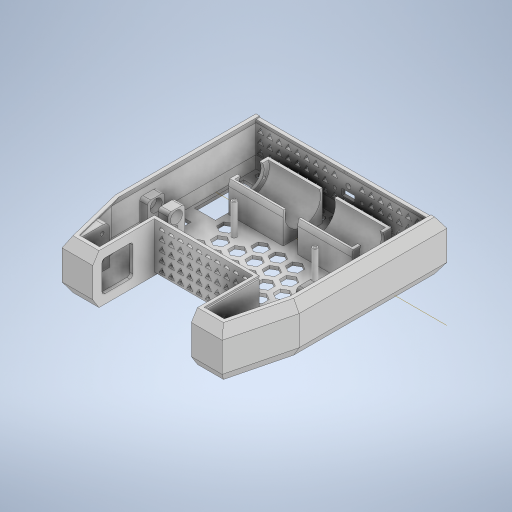
# Autodesk Inventor part: Bot v2 bottom
Saved by Autodesk Inventor 2024 (Build 280153000, 153)
## iProperties
Created: 2023-10-31
Part Number: Bot v2 bottom
Material: Generic
Document SubType Name: Modeling
Designer: CJ110
Density: 1 g/cm^3
Appearance: Default
Mass: 342.153 g
Surface Area: 1832.33 cm^2
Volume: 342.153 cm^3
Author: CJ110
## iProperties of the stored document Bot v2 bottom_3DPrint.ipt
Created: 2023-11-01
Part Number: Bot v2 bottom_3DPrint
Material: Generic
Document SubType Name: Modeling
Designer: CJ110
Density: 1 g/cm^3
Appearance: Default
Author: CJ110
Autodesk Inventor part; units mm, degrees
(part 1 of 3)
sketch "Sketch1" plane through (0, 0, 0) normal (0, 1, 0) x (-1, 0, 0)
  line L0 (0, 0) -> (152.4, 0)
  line L1 (152.4, 0) -> (152.4, 196.85)
  line L2 (152.4, 196.85) -> (0, 196.85)
  line L3 (0, 196.85) -> (0, 0)
  line L4 (152.4, 196.85) -> (215.9, 180.975)
  line L5 (215.9, 180.975) -> (215.9, 149.225)
  line L6 (215.9, 149.225) -> (152.4, 149.225)
  line L7 (152.4, 47.625) -> (215.9, 47.625)
  line L8 (215.9, 47.625) -> (215.9, 15.875)
  line L9 (215.9, 15.875) -> (152.4, 0)
  dimension "Bot_Main_Length" = 152.4
  dimension "Bot_Width" = 196.85
  dimension "Weapon_Support_Depth" = 63.5
  dimension "Weapon_Width" = 101.6
  dimension "d4" = 31.75
  dimension "d5" = 31.75
  constraints: 20 end point, 4 point on line, 3 parallel, 2 perpendicular, 1 equal length, 1 horizontal, 1 vertical
  measures "Bot_Main_Length" distance of L2.end L1.end
  measures "Bot_Width" distance of L0.end L1.end
  measures "Weapon_Support_Depth" distance between parallel lines of L1 L5
  measures "Weapon_Width" distance between parallel lines of L7 L6
  measures "d4" distance of L4.end L5.end
  measures "d5" distance of L7.end L8.end
extrude "Extrusion1" add sketch "Sketch1" along normal blind 50.8
chamfer "Chamfer1" distance 6.35 distance2 10.16 7 edges at (-76.2, 50.8, 196.85) (-184.15, 50.8, 188.9125) (0, 50.8, 98.425) (-76.2, 50.8, 0) (-184.15, 50.8, 7.9375) (-215.9, 50.8, 31.75) (-215.9, 50.8, 165.1) measured on face at (-215.4, 50.8, 165.1) measured on face at (-0.5, 50.8, 98.425) measured on face at (-184.0287, 50.8, 188.4274) measured on face at (-76.2, 50.8, 0.5) measured on face at (-76.2, 50.8, 196.35) measured on face at (-215.4, 50.8, 31.75) measured on face at (-184.0287, 50.8, 8.4226)
chamfer "Chamfer2" distance 6.35 distance2 10.16 7 edges at (-76.2, 0, 196.85) (-184.15, 0, 188.9125) (-215.9, 0, 165.1) (-184.15, 0, 7.9375) (-215.9, 0, 31.75) (-76.2, 0, 0) (0, 0, 98.425) measured on face at (-215.4, 0, 165.1) measured on face at (-184.0287, 0, 188.4274) measured on face at (-76.2, 0, 196.35) measured on face at (-76.2, 0, 0.5) measured on face at (-0.5, 0, 98.425) measured on face at (-184.0287, 0, 8.4226) measured on face at (-215.4, 0, 31.75)
shell "Shell1" thickness 3.175 removed faces 1 at (-55.033333, 50.8, 115.358333)
sketch "Sketch2" plane through (-151.401646, 3.175, 188.740264) normal (0, 1, 0) x (1, 0, 0)
  line L0 (11.701646, 3.175) -> (62.501646, 3.175)
  line L1 (62.501646, 3.175) -> (62.501646, 13.97)
  line L2 (62.501646, 13.97) -> (11.701646, 13.97)
  line L3 (11.701646, 13.97) -> (11.701646, 3.175)
  line L4 (76.61691, 3.175) -> (127.41691, 3.175)
  line L5 (127.41691, 3.175) -> (127.41691, 24.765)
  line L6 (127.41691, 24.765) -> (76.61691, 24.765)
  line L7 (76.61691, 24.765) -> (76.61691, 3.175)
  line L8 (143.29191, 0) -> (143.29191, 180.630527)
  line L9 (0, 0) -> (143.29191, 0)
  line L10 (2.176646, 36.340264) -> (2.176646, 144.290264)
  line L11 (2.176646, 90.315264) -> (141.307535, 90.315264) construction
  line L12 (141.307535, 178.646152) -> (141.307535, 1.984375) construction
  line L13 (-56.388618, 36.340264) -> (-56.388618, 14.097154)
  line L14 (-56.388618, 14.097154) -> (0, 0)
  line L15 (0, 0) -> (143.29191, 0)
  line L16 (143.29191, 0) -> (143.29191, 180.630527)
  line L17 (143.29191, 180.630527) -> (0, 180.630527)
  line L18 (0, 180.630527) -> (-56.388618, 166.533373)
  line L19 (-56.388618, 166.533373) -> (-56.388618, 144.290264)
  line L20 (-56.388618, 144.290264) -> (2.176646, 144.290264)
  line L21 (2.176646, 144.290264) -> (2.176646, 36.340264)
  line L22 (2.176646, 36.340264) -> (-56.388618, 36.340264)
  line L23 (11.701646, 177.455527) -> (62.501646, 177.455527)
  line L24 (62.501646, 177.455527) -> (62.501646, 166.660527)
  line L25 (62.501646, 166.660527) -> (11.701646, 166.660527)
  line L26 (11.701646, 166.660527) -> (11.701646, 177.455527)
  line L27 (76.61691, 177.455527) -> (127.41691, 177.455527)
  line L28 (127.41691, 177.455527) -> (127.41691, 155.865527)
  line L29 (127.41691, 155.865527) -> (76.61691, 155.865527)
  line L30 (76.61691, 155.865527) -> (76.61691, 177.455527)
  line L31 (102.01691, 24.765) -> (102.01691, 3.175) construction
  line L32 (37.101646, 13.97) -> (37.101646, 3.175) construction
  point P0 (151.401646, 188.740264)
  dimension "d15" = 21.59
  dimension "d16" = 50.8
  dimension "d17" = 50.8
  dimension "d19" = 3.175
  dimension "d21" = 10.795
  dimension "d165" = 41.275
  dimension "d166" = 34.925
  constraints: 38 end point, 8 symmetric about line, 6 midpoint, 4 parallel, 2 horizontal, 2 perpendicular, 1 collinear
  measures "d15" distance between parallel lines of L6 L4
  measures "d16" distance between parallel lines of L3 L1
  measures "d17" distance between parallel lines of L7 L5
  measures "d19" distance between parallel lines of L9 L4
  measures "d21" distance between parallel lines of L0 L2
  measures "d165" distance between parallel lines of L31 L8
  measures "d166" distance between parallel lines of L10 L32
extrude "Extrusion2" cut sketch "Sketch2" against normal through all contours L3 L2 L1 L0 | L7 L6 L5 L4 | L23 L24 L25 L26 | L27 L28 L29 L30
sketch "Sketch3" plane through (0, 40.64, 196.85) normal (1, 0, 0) x (0, 0, -1)
  line L0 (190.5, 10.16) -> (6.35, 10.16)
  line L1 (6.35, 10.16) -> (0, 0)
  line L2 (0, 0) -> (196.85, 0)
  line L3 (190.5, 10.16) -> (196.85, 0)
  line L4 (10.094111, 10.16) -> (8.109736, 6.985)
  line L5 (8.109736, 6.985) -> (188.740264, 6.985)
  line L6 (186.755889, 10.16) -> (188.740264, 6.985)
  point P0 (196.85, -40.64)
  dimension "d24" = 3.175
  dimension "d25" = 3.175
  dimension "d26" = 3.175
  constraints: 6 end point, 2 parallel, 2 point on line, 1 horizontal
  measures "d24" distance between parallel lines of L1 L4
  measures "d25" distance between parallel lines of L0 L5
  measures "d26" distance between parallel lines of L3 L6
extrude "Extrusion3" cut sketch "Sketch3" against normal up to surface contours L6 L5 L4 L0 surface through (-5.867395, 44.037253, 147.6375) normal (0.8479983, 0.5299989, 0)
sketch "Sketch4" plane through (-149.225, 3.175, 44.45) normal (1, 0, 0) x (0, 0, -1)
  line L0 (-144.290264, 44.45) -> (-142.305889, 47.625)
  line L1 (-142.305889, 47.625) -> (-146.05, 47.625)
  line L2 (-146.05, 47.625) -> (-152.4, 37.465)
  line L3 (-152.4, 37.465) -> (44.45, 37.465)
  line L4 (38.1, 47.625) -> (44.45, 37.465)
  line L5 (38.1, 47.625) -> (34.355889, 47.625)
  line L6 (34.355889, 47.625) -> (36.340264, 44.45)
  line L7 (36.340264, 44.45) -> (-144.290264, 44.45)
  line L8 (0, 0) -> (-107.95, 0)
  line L9 (0, 0) -> (0, 47.625)
  line L10 (-107.95, 47.625) -> (0, 47.625)
  line L11 (-107.95, 0) -> (-107.95, 47.625)
  line L12 (0, 46.0375) -> (-107.95, 46.0375)
  line L13 (-106.3625, 46.0375) -> (-106.3625, 44.45)
  line L14 (-1.5875, 46.0375) -> (-1.5875, 44.45)
  point P0 (44.45, -3.175)
  point P1 (-107.95, 44.45)
  point P2 (0, 44.45)
  dimension "d29" = 1.5875
  dimension "d30" = 1.5875
  dimension "d31" = 1.5875
  constraints: 6 end point, 6 point on line, 3 perpendicular
  measures "d29" distance between parallel lines of L10 L12
  measures "d30" distance between parallel lines of L11 L13
  measures "d31" distance between parallel lines of L9 L14
extrude "Extrusion4" cut sketch "Sketch4" against normal blind 1.5875 contours L13 L12 L14 L7
extrude "Extrusion5" cut sketch "Sketch4" against normal up to surface contours L11 L12 L13 L7 | L14 L12 L9 L7 surface through (-210.032605, 44.037253, 123.825) normal (-0.8479983, 0.5299989, 0)
sketch "Sketch5" plane through (-151.401646, 3.175, 188.740264) normal (0, 1, 0) x (1, 0, 0)
  line L0 (88.50411, 29.845) -> (129.14411, 29.845)
  line L1 (129.14411, 29.845) -> (129.14411, 82.677)
  line L2 (129.14411, 82.677) -> (88.50411, 82.677)
  line L3 (88.50411, 82.677) -> (88.50411, 29.845)
  line L4 (102.01691, 233.61858) -> (102.01691, -48.397789)
  line L5 (76.61691, 24.765) -> (127.41691, 24.765)
  line L6 (2.176646, 144.290264) -> (2.176646, 36.340264)
  line L7 (2.176646, 90.315264) -> (143.29191, 90.315264) construction
  line L8 (143.29191, 0) -> (143.29191, 180.630527)
  line L9 (88.50411, 150.785527) -> (129.14411, 150.785527)
  line L10 (129.14411, 150.785527) -> (129.14411, 97.953527)
  line L11 (129.14411, 97.953527) -> (88.50411, 97.953527)
  line L12 (88.50411, 97.953527) -> (88.50411, 150.785527)
  line L13 (108.82411, 82.677) -> (108.82411, 29.845) construction
  point P0 (151.401646, 188.740264)
  dimension "d36" = 40.64
  dimension "d38" = 52.832
  dimension "d39" = 5.08
  dimension "d40" = 6.8072
  constraints: 20 end point, 4 midpoint, 4 symmetric about line, 2 parallel, 1 horizontal, 1 perpendicular
  measures "d36" distance between parallel lines of L1 L3
  measures "d38" distance between parallel lines of L2 L0
  measures "d39" distance between parallel lines of L5 L0
  measures "d40" distance between parallel lines of L13 L4
extrude "Extrusion6" add sketch "Sketch5" along normal blind 31.75
ref_plane "Work Plane1" through (-152.4, 40.64, 98.425) normal (0, 0, 1) x (1, 0, 0)
sketch "Sketch6" plane through (-152.4, 40.64, 98.425) normal (0, 0, 1) x (1, 0, 0)
  line L0 (130.142464, -37.465) -> (89.502464, -37.465)
  line L1 (130.142464, -37.465) -> (130.142464, -5.715)
  line L2 (89.502464, -5.715) -> (130.142464, -5.715)
  line L3 (89.502464, -37.465) -> (89.502464, -5.715)
  arc A0 (92.536929, -5.715) -> (127.107999, -5.715) centre (109.822464, -12.065) ccw
  line L4 (130.142464, -5.715) -> (89.502464, -5.715)
  line L5 (109.822464, -5.715) -> (109.822464, -37.465) construction
  arc A1 (130.142464, -8.255) -> (129.497219, -5.715) centre (109.822464, -12.065) ccw
  arc A2 (90.520135, -5.715) -> (89.502464, -12.065) centre (109.822464, -12.065) ccw
  point P0 (152.4, -40.64)
  point P1 (127.107999, -5.715)
  point P2 (129.497219, -5.715)
  point P3 (90.520135, -5.715)
  dimension "d46" = 25.4
  dimension "d47" = 36.83
  constraints: 7 point on line, 6 point on circle, 3 centre point, 2 end point, 2 midpoint, 1 coincident, 1 tangent
  measures "d46" distance from line of L0 A0.centre
  measures "d47" diameter of A0
extrude "Extrusion7" cut sketch "Sketch6" along normal mid plane 142.24 contours L3 L2 A2 | A0 L2
sketch "Sketch7" plane through (-62.897536, 3.175, 158.895264) normal (0, 0, 1) x (1, 0, 0)
  arc A0 (3.034465, 31.75) -> (37.605535, 31.75) centre (20.32, 25.4) ccw
  line L0 (1.017671, 31.75) -> (3.034465, 31.75)
  arc A1 (1.017671, 31.75) -> (0, 25.4) centre (20.32, 25.4) ccw
  line L1 (0, 0) -> (0, 25.4)
  line L2 (40.64, 0) -> (0, 0)
  line L3 (40.64, 0) -> (40.64, 31.75)
  line L4 (37.605535, 31.75) -> (40.64, 31.75)
  circle A2 centre (20.32, 9.906) radius 1.143
  line L5 (20.32, 25.4) -> (20.32, 8.763) construction
  line L6 (11.729879, 6.985) -> (28.910121, 6.985) construction
  circle A3 centre (33.738198, 17.653) radius 1.143
  circle A4 centre (33.738198, 33.147) radius 1.143
  circle A5 centre (20.32, 40.894) radius 1.143
  circle A6 centre (6.901802, 33.147) radius 1.143
  circle A7 centre (6.901802, 17.653) radius 1.143
  line L7 (19.511777, 10.714223) -> (20.32, 11.522446)
  line L8 (20.32, 11.522446) -> (21.128223, 10.714223)
  line L9 (32.929975, 18.461223) -> (33.738198, 19.269446)
  line L10 (33.738198, 19.269446) -> (34.546421, 18.461223)
  arc A8 (1.017671, 31.75) -> (0, 25.4) centre (20.32, 25.4) ccw
  line L11 (0, 0) -> (0, 25.4)
  line L12 (40.64, 0) -> (0, 0)
  line L13 (40.64, 0) -> (40.64, 31.75)
  line L14 (37.605535, 31.75) -> (40.64, 31.75)
  arc A9 (3.034465, 31.75) -> (37.605535, 31.75) centre (20.32, 25.4) ccw
  line L15 (1.017671, 31.75) -> (3.034465, 31.75)
  circle A10 centre (20.32, 25.4) radius 18.415
  circle A11 centre (20.32, 25.4) radius 13.081
  circle A12 centre (20.32, 10.287) radius 1.524
  line L16 (20.32, 25.4) -> (20.32, 8.763) construction
  circle A13 centre (33.408242, 17.8435) radius 1.524
  circle A14 centre (33.408242, 32.9565) radius 1.524
  circle A15 centre (20.32, 40.513) radius 1.524
  circle A16 centre (7.231758, 32.9565) radius 1.524
  circle A17 centre (7.231758, 17.8435) radius 1.524
  line L17 (3.034465, 31.75) -> (37.605535, 31.75)
  point P0 (62.897536, -3.175)
  point P1 (34.728065, 17.0815)
  point P2 (34.728065, 33.7185)
  point P3 (20.32, 42.037)
  point P4 (5.911935, 33.7185)
  point P5 (5.911935, 17.0815)
  point P6 (20.32, 6.985)
  point P7 (34.728065, 17.0815)
  point P8 (34.728065, 33.7185)
  point P9 (20.32, 42.037)
  point P10 (5.911935, 33.7185)
  point P11 (5.911935, 17.0815)
  point P12 (37.605535, 31.75)
  point P13 (33.335423, 38.427317)
  point P14 (32.689677, 39.041969)
  point P15 (7.950323, 39.041969)
  point P16 (7.304577, 38.427317)
  point P17 (3.034465, 31.75)
  point P18 (0, 25.4)
  point P19 (40.64, 31.75)
  point P20 (28.689189, 15.34668)
  point P21 (11.950811, 15.34668)
  point P22 (33.400465, 25.281714)
  point P23 (33.179988, 23.005578)
  point P24 (8.883652, 31.75)
  point P25 (31.756348, 31.75)
  dimension "d160" = 3.048
  dimension "d51" = 2.286
  dimension "d52" = 1.778
  dimension "d55" = 360
  dimension "d157" = 36.83
  dimension "d158" = 5.334
  dimension "d159" = 1.778
  dimension "d163" = 360
  constraints: 16 end point, 7 point on circle, 5 tangent, 5 vertical alignment, 4 centre point, 2 coincident, 2 horizontal, 2 perpendicular, 1 point on line, 1 vertical, 65 other
  measures "d51" diameter of A2
  measures "d52" distance from line of L6 L5.end
  measures "d157" diameter of A10
  measures "d158" radial gap between concentric circles of A10 A11
  measures "d159" distance of point (20.32, 6.985) L16.end
extrude "Extrusion8" add sketch "Sketch7" along normal blind 3.175 contours L17 A16 A11 A14 A0 | A0 L4 L3 L2 L1 A1 L0 | L17 A16 | A14 L17 picked at (7.016219, 31.692159) picked at (33.623781, 31.692159)
mirror "Mirror1" about plane through (-152.4, 40.64, 98.425) normal (0, 0, 1) of "Extrusion8"
sketch "Sketch12" plane through (-152.4, 0, 47.625) normal (0, 0, 1) x (1, 0, 0)
  line L0 (-54.767, 47.879) -> (-21.433, 47.879)
  line L1 (-21.433, 47.879) -> (-21.433, 3.175)
  line L2 (-21.433, 3.175) -> (-55.390264, 3.175)
  line L3 (-54.767, 2.177778) -> (-54.767, 47.879)
  line L4 (-38.1, 47.879) -> (-38.1, 3.175) construction
  line L5 (-63.5, 10.16) -> (-63.5, 40.64)
  line L6 (-55.390264, 3.175) -> (0.998354, 3.175)
  line L7 (0.998354, 3.175) -> (144.290264, 3.175)
  line L8 (144.290264, 3.175) -> (0.998354, 3.175)
  line L9 (0.998354, 3.175) -> (-55.390264, 3.175)
  line L10 (-55.390264, 3.175) -> (3.175, 3.175)
  line L11 (3.175, 3.175) -> (-55.390264, 3.175)
  line L12 (12.7, 3.175) -> (63.5, 3.175)
  line L13 (63.5, 3.175) -> (12.7, 3.175)
  line L14 (128.415264, 3.175) -> (77.615264, 3.175)
  line L15 (77.615264, 3.175) -> (128.415264, 3.175)
  line L16 (12.7, 3.175) -> (63.5, 3.175)
  line L17 (63.5, 3.175) -> (12.7, 3.175)
  line L18 (130.142464, 3.175) -> (89.502464, 3.175)
  line L19 (89.502464, 3.175) -> (130.142464, 3.175)
  line L20 (-55.390264, 3.175) -> (-60.325, 11.070578)
  line L21 (-55.390264, 3.175) -> (-60.325, 11.070578)
  line L22 (89.502464, 3.175) -> (130.142464, 3.175)
  line L23 (130.142464, 3.175) -> (89.502464, 3.175)
  line L24 (77.615264, 3.175) -> (128.415264, 3.175)
  line L25 (128.415264, 3.175) -> (77.615264, 3.175)
  point P0 (152.4, 0)
  point P1 (-38.1, 31.75)
  point P2 (-38.1, 31.75)
  point P3 (-54.767, 12.337778)
  point P4 (-54.767, 3.175)
  dimension "d80" = 33.334
  dimension "d81" = 25.4
  dimension "d83" = 44.704
  constraints: 10 end point, 3 point on line, 2 parallel, 1 coincident, 1 collinear, 1 horizontal, 1 midpoint, 1 perpendicular
  measures "d80" distance between parallel lines of L1 L3
  measures "d81" distance between parallel lines of L5 L4
  measures "d83" distance between parallel lines of L2 L0
extrude "Extrusion12" [suppressed]
fillet "Fillet1" [suppressed]
sketch "Sketch13" plane through (-152.4, 0, 47.625) normal (0, 0, 1) x (1, 0, 0)
  line L0 (-38.1, 47.879) -> (-38.1, 3.175) construction
  line L1 (-57.15, 0) -> (-63.5, 10.16)
  line L2 (-57.15, 0) -> (0, 0)
  line L3 (0, 0) -> (0, 50.8)
  line L4 (-57.15, 50.8) -> (0, 50.8)
  line L5 (-63.5, 40.64) -> (-57.15, 50.8)
  line L6 (-63.5, 10.16) -> (-63.5, 40.64)
  line L7 (-21.433, 3.175) -> (-49.040264, 3.175)
  line L8 (-33.274, 3.175) -> (-34.2265, 5.715)
  line L9 (-34.2265, 5.715) -> (-24.7015, 5.715)
  line L10 (-24.7015, 5.715) -> (-25.654, 3.175)
  line L11 (-45.339, 3.175) -> (-46.2915, 5.715)
  line L12 (-46.2915, 5.715) -> (-36.7665, 5.715)
  line L13 (-36.7665, 5.715) -> (-37.719, 3.175)
  line L14 (-37.854636, 3.175) -> (-36.949761, 5.588)
  line L15 (-36.949761, 5.588) -> (-46.108239, 5.588)
  line L16 (-46.108239, 5.588) -> (-45.203364, 3.175)
  line L17 (-25.789636, 3.175) -> (-24.884761, 5.588)
  line L18 (-24.884761, 5.588) -> (-34.043239, 5.588)
  line L19 (-34.043239, 5.588) -> (-33.138364, 3.175)
  point P0 (152.4, 0)
  point P1 (-29.464, 5.715)
  point P2 (-41.529, 5.715)
  dimension "d87" = 8.636
  dimension "d88" = 7.62
  dimension "d89" = 2.54
  dimension "d90" = 9.525
  dimension "d93" = 0.127
  dimension "d94" = 0.127
  dimension "d95" = 0.127
  dimension "d96" = 0.127
  dimension "d97" = 0.127
  dimension "d98" = 0.127
  dimension "d131" = 12.065
  constraints: 26 end point, 4 equal length, 2 horizontal, 2 midpoint, 1 collinear, 1 vertical, 9 other
  measures "d87" distance from line of L0 point (-29.464, 5.715)
  measures "d88" distance of L10.end L8.start
  measures "d90" distance of L9.end L8.end
  measures "d93" distance between parallel lines of L12 L15
  measures "d94" distance between parallel lines of L9 L18
  measures "d95" distance between parallel lines of L8 L19
  measures "d96" distance between parallel lines of L10 L17
  measures "d97" distance between parallel lines of L13 L14
  measures "d98" distance between parallel lines of L11 L16
  measures "d131" distance of point (-41.529, 5.715) point (-29.464, 5.715)
extrude "Extrusion13" [suppressed]
sketch "Sketch15" plane through (-212.725, 11.070578, 44.45) normal (0, 0, -1) x (-1, 0, 0)
  line L0 (-4.934736, -7.895578) -> (0, 0)
  line L1 (0, 0) -> (0, 28.658844)
  line L2 (0, 28.658844) -> (-4.934736, 36.554422)
  line L3 (-4.934736, 36.554422) -> (-63.5, 36.554422)
  line L4 (-63.5, -7.895578) -> (-63.5, 36.554422)
  line L5 (-4.934736, -7.895578) -> (-63.5, -7.895578)
  line L6 (-32.542, -7.895578) -> (-40.289, 5.52262)
  line L7 (-40.289, 5.52262) -> (-40.289, 13.26962)
  line L8 (-40.289, 13.26962) -> (-32.542, 13.26962)
  circle A0 centre (-42.5704, 2.772422) radius 1.5875
  line L9 (-40.289, 5.52262) -> (-40.289, -7.895578)
  line L10 (-32.542, 13.26962) -> (-40.289, 13.26962)
  line L11 (3.175, -0.910578) -> (3.175, 29.569422)
  line L12 (3.175, 14.329422) -> (-38.892, 14.329422) construction
  point P0 (-212.725, -11.070578)
  point P1 (-22.225, 30.458422)
  point P2 (-32.542, -7.895578)
  dimension "d107" = 7.747
  dimension "d108" = 7.747
  dimension "d110" = 3.175
  dimension "d122" = 20.3454
  dimension "d136" = 11.557
  constraints: 12 end point, 1 centre point, 1 horizontal, 1 midpoint, 1 perpendicular, 1 point on line, 1 vertical
  measures "d107" distance of L7.end L8.end
  measures "d108" distance of L6.end L7.end
  measures "d110" diameter of A0
  measures "d122" horizontal distance of A0.centre point (-22.225, 30.458)
  measures "d136" distance from line of L12 A0.centre
extrude "Extrusion14" [suppressed]
fillet "Fillet2" [suppressed]
extrude "Extrusion15" [suppressed]
fillet "Fillet3" [suppressed]
sketch "Sketch16" plane through (-152.4, 0, 149.225) normal (0, 0, -1) x (-1, 0, 0)
  circle A0 centre (38.1, 25.4) radius 7.0485
  line L0 (63.5, 10.16) -> (63.5, 40.64) projected
  line L1 (63.5, 25.4) -> (0, 25.4) construction
  line L2 (0, 0) -> (0, 50.8) projected
  line L3 (63.5, 10.16) -> (57.15, 0) projected
  line L4 (63.5, 10.16) -> (63.5, 40.64) projected
  line L5 (57.15, 50.8) -> (63.5, 40.64) projected
  line L6 (0, 50.8) -> (57.15, 50.8) projected
  line L7 (0, 0) -> (0, 50.8) projected
  line L8 (0, 0) -> (57.15, 0) projected
  point P0 (-152.4, 0)
  dimension "d137" = 14.097
  dimension "d201" = 38.1
  constraints: 3 midpoint, 2 end point, 1 centre point, 1 point on line
  measures "d137" diameter of A0
  measures "d201" distance of A0.centre point (0, 25.4)
hole "Hole1" [suppressed]
sketch "Sketch17" plane through (-166.086, 16.593198, 53.975) normal (1, 0, 0) x (0, 0, -1)
  line L0 (9.525, -13.418198) -> (9.525, -5.52262)
  line L1 (9.525, -5.52262) -> (9.525, 23.136224)
  line L2 (9.525, 23.136224) -> (9.525, 31.031802)
  line L3 (9.525, -13.418198) -> (9.525, 31.031802)
  line L4 (3.175, 7.747) -> (3.175, -13.418198)
  line L5 (0, 7.747) -> (3.175, 7.747)
  line L6 (0, 4.572) -> (0, 7.747)
  line L7 (0, 0) -> (0, 4.572)
  line L8 (0, -13.418198) -> (0, 0)
  line L9 (3.175, 7.747) -> (0, 14.097)
  line L10 (3.175, -13.418198) -> (0, -13.418198)
  point P0 (53.975, -16.593198)
  point P1 (9.525, 31.031802)
  dimension "d133" = 6.35
  constraints: 2 end point, 2 other
  measures "d133" distance from line of L5 L9.end
extrude "Extrusion16" [suppressed]
extrude "Extrusion17" cut sketch "Sketch16" against normal up to surface (3.175 mm away) contours A0
ref_plane "Work Plane3" through (0, 25.4, 0) normal (0, 1, 0) x (-1, 0, 0)
sketch "Sketch18" plane through (0, 25.4, 0) normal (0, 1, 0) x (-1, 0, 0)
  line L0 (139.7, 11.284736) -> (88.9, 11.284736)
  line L1 (114.3, 11.284736) -> (114.3, 185.565264) construction
  line L2 (139.7, 185.565264) -> (88.9, 185.565264)
  line L3 (88.9, 22.079736) -> (139.7, 22.079736)
  line L4 (123.063, 22.079736) -> (105.537, 22.079736)
  line L5 (105.537, 22.079736) -> (105.537, 32.239736)
  line L6 (105.537, 32.239736) -> (123.063, 32.239736)
  line L7 (123.063, 32.239736) -> (123.063, 22.079736)
  line L8 (152.00914, 3.175) -> (3.175, 3.175)
  line L9 (3.175, 3.175) -> (152.00914, 3.175)
  line L10 (123.063, 3.175) -> (105.537, 3.175)
  line L11 (105.537, 3.175) -> (105.537, 11.284736)
  line L12 (105.537, 11.284736) -> (123.063, 11.284736)
  line L13 (123.063, 11.284736) -> (123.063, 3.175)
  point P0 (0, 0)
  point P1 (105.537, 22.079736)
  point P2 (123.063, 3.175)
  point P3 (123.063, 11.284736)
  point P4 (105.537, 3.175)
  point P5 (17.634736, 17.634736)
  point P6 (17.634736, 198.265264)
  point P7 (93.834736, 28.429736)
  point P8 (105.537, 22.079736)
  point P9 (123.063, 11.284736)
  point P10 (88.9, 28.429736)
  dimension "d141" = 17.526
  dimension "d143" = 8.763
  dimension "d147" = 10.16
  constraints: 18 end point, 4 parallel, 2 collinear, 2 horizontal, 2 perpendicular, 1 point on line, 7 other
  measures "d141" distance between parallel lines of L7 L5
  measures "d143" distance between parallel lines of L1 L7
  measures "d147" distance between parallel lines of L6 L4
extrude "Extrusion18" add sketch "Sketch18" against normal up to next
extrude "Extrusion19" add sketch "Sketch18" along normal blind 7.62
sketch "Sketch19" plane through (-123.063, 25.4, 32.239736) normal (0, 0, 1) x (1, 0, 0)
  line L0 (-136.525, 0) -> (169.291, 0) projected
  line L1 (0, 7.62) -> (17.526, 7.62) projected
  line L2 (8.763, 7.62) -> (8.763, -22.225) construction
  line L3 (17.526, -22.225) -> (0, -22.225) projected
  circle A0 centre (8.763, 0) radius 6.223
  point P0 (123.063, -25.4)
  dimension "d150" = 12.446
  constraints: 2 end point, 2 midpoint, 2 point on line, 1 centre point
  measures "d150" diameter of A0
extrude "Extrusion20" cut sketch "Sketch19" against normal blind 26.67
sketch "Sketch21" plane through (-123.063, 3.175, 32.239736) normal (0, 0, 1) x (1, 0, 0)
  circle A0 centre (8.763, 13.335) radius 1.524
  circle A1 centre (8.763, 22.225) radius 6.223
  line L0 (8.763, 22.225) -> (8.763, 0) construction
  line L1 (0, 0) -> (-16.637, 0)
  line L2 (-16.637, 0) -> (0, 0)
  line L3 (0, 0) -> (-28.338646, 0)
  line L4 (-28.338646, 0) -> (-84.727264, 0)
  line L5 (-84.727264, 0) -> (-26.162, 0)
  line L6 (-26.162, 0) -> (-84.727264, 0)
  line L7 (-84.727264, 0) -> (-28.338646, 0)
  line L8 (-28.338646, 0) -> (114.953264, 0)
  line L9 (114.953264, 0) -> (17.526, 0)
  line L10 (17.526, 0) -> (34.163, 0)
  line L11 (48.278264, 0) -> (99.078264, 0)
  line L12 (99.078264, 0) -> (48.278264, 0)
  line L13 (-16.637, 0) -> (34.163, 0)
  line L14 (34.163, 0) -> (-16.637, 0)
  circle A2 centre (8.763, 22.225) radius 6.223
  line L15 (17.526, 0) -> (0, 0)
  line L16 (17.526, 29.845) -> (17.526, 0)
  line L17 (0, 29.845) -> (17.526, 29.845)
  line L18 (0, 0) -> (0, 29.845)
  line L19 (60.165464, 0) -> (100.805464, 0)
  line L20 (100.805464, 0) -> (60.165464, 0)
  line L21 (100.805464, 0) -> (60.165464, 0)
  line L22 (60.165464, 0) -> (100.805464, 0)
  line L23 (99.078264, 0) -> (48.278264, 0)
  line L24 (17.526, 0) -> (0, 0)
  line L25 (34.163, 0) -> (17.526, 0)
  line L26 (48.278264, 0) -> (99.078264, 0)
  point P0 (123.063, -3.175)
  dimension "d153" = 3.048
  dimension "d154" = 8.89
  constraints: 2 end point, 1 centre point, 1 midpoint, 1 point on line, 1 vertical
  measures "d153" diameter of A0
  measures "d154" distance of A0.centre L0.start
extrude "Extrusion21" cut sketch "Sketch21" against normal up to surface (10.16 mm away) contours A0
mirror "Mirror2" about plane through (-152.4, 40.64, 98.425) normal (0, 0, 1) of "Extrusion18", "Extrusion19", "Extrusion20", "Extrusion21"
sketch "Sketch22" plane through (-207.790264, 3.175, 152.4) normal (0, 0, 1) x (1, 0, 0)
  line L0 (16.020264, 15.8115) -> (18.560264, 15.8115)
  line L1 (18.560264, 15.8115) -> (18.560264, 13.2715)
  line L2 (18.560264, 13.2715) -> (16.020264, 13.2715)
  line L3 (16.020264, 13.2715) -> (16.020264, 15.8115)
  circle A0 centre (17.290264, 22.225) radius 7.0485
  line L4 (17.290264, 29.2735) -> (17.290264, 15.1765) construction
  point P0 (207.790264, -3.175)
  dimension "d168" = 2.54
  dimension "d169" = 1.27
  dimension "d170" = 1.905
  dimension "d171" = 0.635
  constraints: 10 end point, 2 parallel, 2 point on circle, 1 horizontal, 1 midpoint, 1 perpendicular, 1 vertical
  measures "d168" distance between parallel lines of L1 L3
  measures "d169" distance between parallel lines of L4 L3
  measures "d170" distance from line of L4.end L2
  measures "d171" distance from line of L4.end L0
extrude "Extrusion22" add sketch "Sketch22" along normal blind 1.27 contours L0 L1 A0 L3 | A0 L1 L2 L3 picked at (17.432064, 15.604116)
chamfer "Chamfer4" distance 1.27 distance2 2.54 1 edges at (-190.5, 16.4465, 153.67) measured on face at (-190.5, 16.4465, 153.17)
sketch "Sketch23" plane through (-207.790264, 3.175, 152.4) normal (0, 0, 1) x (1, 0, 0)
  arc A0 (18.560264, 15.291858) -> (16.020264, 15.291858) centre (17.290264, 22.225) ccw
  circle A1 centre (17.290264, 22.225) radius 5.08
  line L0 (10.241764, 29.2735) -> (24.338764, 29.2735)
  line L1 (24.338764, 29.2735) -> (24.338764, 13.2715)
  line L2 (24.338764, 13.2715) -> (10.241764, 13.2715)
  line L3 (10.241764, 13.2715) -> (10.241764, 29.2735)
  line L4 (18.560264, 13.2715) -> (16.020264, 13.2715)
  point P0 (207.790264, -3.175)
  dimension "d177" = 10.16
  constraints: 8 end point, 3 tangent, 2 parallel, 1 centre point, 1 coincident, 1 collinear, 1 horizontal, 1 perpendicular
  measures "d177" diameter of A1
extrude "Extrusion23" add sketch "Sketch23" along normal blind 1.27
chamfer "Chamfer5" distance 3.81 distance2 1.27 1 edges at (-190.5, 16.4465, 153.67) measured on face at (-190.5, 16.9465, 153.67)
chamfer "Chamfer6" distance 3.81 distance2 1.27 1 edges at (-183.4515, 32.4485, 153.035) measured on face at (-183.4515, 31.9485, 153.035)
chamfer "Chamfer7" distance 3.81 distance2 1.27 1 edges at (-197.5485, 32.4485, 153.035) measured on face at (-197.5485, 31.9485, 153.035)
sketch "Sketch24" plane through (-152.4, 0, 47.625) normal (0, 0, 1) x (1, 0, 0)
  line L0 (-54.102, 41.402) -> (-22.098, 41.402)
  line L1 (-22.098, 41.402) -> (-22.098, 9.398)
  line L2 (-22.098, 9.398) -> (-54.102, 9.398)
  line L3 (-54.102, 9.398) -> (-54.102, 41.402)
  circle A0 centre (-38.1, 25.4) radius 7.0485 projected
  arc A1 (-45.1485, 25.4) -> (-31.0515, 25.4) centre (-38.1, 25.4) ccw projected
  arc A2 (-31.0515, 25.4) -> (-38.1, 32.4485) centre (-38.1, 25.4) ccw projected
  arc A3 (-38.1, 32.4485) -> (-45.1485, 25.4) centre (-38.1, 25.4) ccw projected
  line L4 (-38.1, 41.402) -> (-38.1, 9.398) construction
  line L5 (-22.098, 25.4) -> (-54.102, 25.4) construction
  point P0 (152.4, 0)
  dimension "d189" = 32.004
  dimension "d190" = 32.004
  constraints: 12 end point, 6 midpoint, 2 parallel, 1 horizontal, 1 perpendicular
  measures "d189" distance between parallel lines of L2 L0
  measures "d190" distance between parallel lines of L1 L3
extrude "Extrusion24" cut sketch "Sketch24" against normal up to surface (3.175 mm away) contours L0 L1 L2 L3 | A0
fillet "Fillet4" radius 3.175 4 edges at (-174.498, 41.402, 46.0375) (-174.498, 9.398, 46.0375) (-206.502, 9.398, 46.0375) (-206.502, 41.402, 46.0375)
ref_plane "Work Plane4" through (-149.225, 3.175, 20.32) normal (0, 0, -1) x (-1, 0, 0)
sketch "Sketch26" plane through (-149.225, 3.175, 20.32) normal (0, 0, -1) x (-1, 0, 0)
  line L0 (28.448, 6.223) -> (54.102, 6.223)
  arc A0 (54.102, 6.223) -> (57.277, 9.398) centre (54.102, 9.398) ccw
  line L1 (57.277, 9.398) -> (57.277, 35.052)
  arc A1 (57.277, 35.052) -> (54.102, 38.227) centre (54.102, 35.052) ccw
  line L2 (54.102, 38.227) -> (28.448, 38.227)
  arc A2 (28.448, 38.227) -> (25.273, 35.052) centre (28.448, 35.052) ccw
  line L3 (25.273, 35.052) -> (25.273, 9.398)
  arc A3 (25.273, 9.398) -> (28.448, 6.223) centre (28.448, 9.398) ccw
  line L4 (60.325, -3.175) -> (66.675, 6.985)
  line L5 (60.325, -3.175) -> (3.175, -3.175)
  line L6 (3.175, -3.175) -> (3.175, 47.625)
  line L7 (60.325, 47.625) -> (3.175, 47.625)
  line L8 (66.675, 37.465) -> (60.325, 47.625)
  line L9 (66.675, 6.985) -> (66.675, 37.465)
  line L10 (63.5, 7.895578) -> (63.5, 36.554422)
  line L11 (63.5, 7.895578) -> (63.5, 36.554422)
  line L12 (56.580889, 47.625) -> (63.5, 36.554422)
  line L13 (57.573076, 46.0375) -> (56.580889, 47.625)
  line L14 (57.573076, 46.0375) -> (58.565264, 44.45)
  line L15 (63.5, 36.554422) -> (58.565264, 44.45)
  line L16 (58.565264, 0) -> (63.5, 7.895578)
  line L17 (58.565264, 0) -> (63.5, 7.895578)
  line L18 (56.580889, 47.625) -> (1.932358, 47.625)
  line L19 (56.580889, 47.625) -> (63.5, 36.554422)
  line L20 (2.78414, 36.554422) -> (63.5, 36.554422)
  line L21 (1.932358, 47.625) -> (2.78414, 36.554422)
  line L22 (63.5, 7.895578) -> (2.78414, 7.895578)
  line L23 (58.565264, 0) -> (63.5, 7.895578)
  line L24 (2.176646, 0) -> (58.565264, 0)
  line L25 (2.176646, 0) -> (2.78414, 7.895578)
  line L26 (28.448, 41.402) -> (54.102, 41.402)
  arc A4 (60.452, 35.052) -> (54.102, 41.402) centre (54.102, 35.052) ccw
  line L27 (60.452, 35.052) -> (60.452, 3.018778)
  line L28 (22.098, 0) -> (22.098, 35.052)
  arc A5 (28.448, 41.402) -> (22.098, 35.052) centre (28.448, 35.052) ccw
  point P0 (-149.225, -3.175)
  point P1 (60.452, 3.018778)
  dimension "d202" = 3.175
  dimension "d203" = 3.175
  dimension "d204" = 3.175
  dimension "d205" = 3.175
  constraints: 6 end point, 4 point on circle, 2 centre point, 2 point on line, 1 other
  measures "d202" distance between parallel lines of L2 L26
  measures "d203" distance between parallel lines of L28 L3
  measures "d204" distance between parallel lines of L1 L27
  measures "d205" radial gap between concentric circles of A2 A5
extrude "Extrusion26" add sketch "Sketch26" along normal up to next contours A3 L22 A0 L0 | L0 A0 L22 L27 L16 L24 L28 A3 | L22 L28 A5 L20 A2 L3 A3 | A3 L3 A2 L20 A1 L1 A0 L22 | A0 L1 A1 L20 A4 L27 L22 | L20 A5 L26 A4 A1 L2 A2 | A2 L2 A1 L20
sketch "Sketch27" plane through (-149.225, 3.175, 20.32) normal (0, 0, 1) x (1, 0, 0)
  circle A0 centre (-52.815, 10.685) radius 2
  circle A1 centre (-52.815, 33.765) radius 2
  circle A2 centre (-29.735, 33.765) radius 2
  circle A3 centre (-29.735, 10.685) radius 2
  line L0 (-54.102, 41.402) -> (-28.448, 41.402)
  line L1 (-41.275, 41.402) -> (-41.275, 0) construction
  line L2 (-22.098, 0) -> (-51.017701, 0)
  line L3 (-28.448, 6.223) -> (-54.102, 6.223)
  arc A4 (-57.277, 9.398) -> (-54.102, 6.223) centre (-54.102, 9.398) ccw
  line L4 (-57.277, 9.398) -> (-57.277, 35.052)
  arc A5 (-54.102, 38.227) -> (-57.277, 35.052) centre (-54.102, 35.052) ccw
  line L5 (-54.102, 38.227) -> (-28.448, 38.227)
  arc A6 (-25.273, 35.052) -> (-28.448, 38.227) centre (-28.448, 35.052) ccw
  line L6 (-25.273, 35.052) -> (-25.273, 9.398)
  arc A7 (-28.448, 6.223) -> (-25.273, 9.398) centre (-28.448, 9.398) ccw
  line L7 (-60.325, -3.175) -> (-66.675, 6.985)
  line L8 (-60.325, -3.175) -> (-3.175, -3.175)
  line L9 (-3.175, -3.175) -> (-3.175, 47.625)
  line L10 (-60.325, 47.625) -> (-3.175, 47.625)
  line L11 (-66.675, 37.465) -> (-60.325, 47.625)
  line L12 (-66.675, 6.985) -> (-66.675, 37.465)
  line L13 (-109.855, 22.225) -> (192.405, 22.225)
  point P0 (149.225, -3.175)
  dimension "d208" = 23.08
  dimension "d209" = 23.08
  dimension "d210" = 11.54
  dimension "d211" = 11.54
  dimension "d212" = 4
  constraints: 4 centre point, 3 equal radius, 2 end point, 2 horizontal alignment, 2 vertical alignment, 1 midpoint, 1 point on line, 1 vertical
  measures "d208" distance of A1.centre A2.centre
  measures "d209" distance of A3.centre A2.centre
  measures "d210" distance from line of L1 A2.centre
  measures "d211" distance from line of A2.centre L13
  measures "d212" diameter of A0
extrude "Extrusion27" cut sketch "Sketch27" against normal blind 4.5 contours A0 | A1 | A2 | A3
sketch "Sketch28" plane through (0, 40.64, 196.85) normal (1, 0, 0) x (0, 0, -1)
  circle A0 centre (98.425, 3.81) radius 1.5875
  line L0 (150.8125, 6.985) -> (46.0375, 6.985) projected
  line L1 (98.425, 6.985) -> (98.425, -40.64) construction
  line L2 (6.35, -40.64) -> (190.5, -40.64) projected
  point P0 (196.85, -40.64)
  dimension "d215" = 3.175
  dimension "d216" = 3.175
  constraints: 2 end point, 2 midpoint, 1 centre point, 1 point on line, 1 vertical
  measures "d215" distance from line of L0 A0.centre
  measures "d216" diameter of A0
extrude "Extrusion28" cut sketch "Sketch28" against normal up to surface surface through (-5.867395, 44.037253, 147.6375) normal (0.8479983, 0.5299989, 0)
sketch "Sketch29" plane through (-207.790264, 3.175, 44.45) normal (0, 1, 0) x (1, 0, 0)
  line L0 (1.984375, -107.95) -> (58.565264, -107.95)
  line L1 (78.885264, -116.985264) -> (78.885264, -120.160264)
  line L2 (78.885264, -120.160264) -> (58.565264, -120.160264)
  line L3 (58.565264, -120.160264) -> (55.390264, -120.160264)
  line L4 (55.390264, -120.160264) -> (55.390264, -107.95)
  line L5 (55.390264, -3.175) -> (55.390264, -104.775)
  line L6 (58.565264, -107.95) -> (58.565264, -116.985264)
  line L7 (58.565264, -116.985264) -> (78.885264, -116.985264)
  line L8 (58.565264, -107.95) -> (58.565264, 0)
  line L9 (58.565264, -90.950264) -> (78.885264, -90.950264)
  line L10 (78.885264, -90.950264) -> (78.885264, -94.125264)
  line L11 (78.885264, -94.125264) -> (58.565264, -94.125264)
  line L12 (58.565264, -94.125264) -> (58.565264, -90.950264)
  line L13 (129.177264, -99.205264) -> (132.352264, -99.205264)
  line L14 (132.352264, -99.205264) -> (132.352264, -111.905264)
  line L15 (132.352264, -111.905264) -> (129.177264, -111.905264)
  line L16 (129.177264, -111.905264) -> (129.177264, -99.205264)
  line L17 (58.565264, -105.555264) -> (129.177264, -105.555264) construction
  line L18 (84.727264, -120.160264) -> (102.253264, -120.160264)
  point P0 (207.790264, 44.45)
  point P1 (58.565264, -94.125264)
  dimension "d219" = 22.86
  dimension "d220" = 3.175
  dimension "d221" = 20.32
  dimension "d222" = 3.175
  dimension "d224" = 3.175
  dimension "d225" = 12.7
  dimension "d226" = 11.43
  dimension "d227" = 70.612
  dimension "d260" = 0
  constraints: 30 end point, 5 perpendicular, 4 horizontal, 4 parallel, 4 point on line, 2 collinear, 2 midpoint, 2 vertical
  measures "d219" distance between parallel lines of L7 L11
  measures "d220" distance between parallel lines of L11 L9
  measures "d221" distance between parallel lines of L8 L10
  measures "d222" distance between parallel lines of L7 L2
  measures "d224" distance between parallel lines of L14 L16
  measures "d225" distance of L13.end L14.end
  measures "d226" distance between parallel lines of L17 L11
  measures "d227" distance between parallel lines of L16 L8
  measures "d260" distance between parallel lines of L18 L2
extrude "Extrusion29" [suppressed]
sketch "Sketch30" plane through (-78.613, 3.175, 143.655264) normal (-1, 0, 0) x (0, 0, 1)
  circle A0 centre (6.35, 17.145) radius 1.5875
  line L0 (0, 0) -> (12.7, 0) projected
  line L1 (0, 0) -> (0, 20.32) projected
  line L2 (12.7, 20.32) -> (0, 20.32) projected
  line L3 (12.7, 0) -> (12.7, 20.32) projected
  line L4 (6.35, 20.32) -> (6.35, 0) construction
  point P0 (-143.655264, -3.175)
  dimension "d230" = 3.175
  dimension "d231" = 3.175
  constraints: 2 end point, 2 midpoint, 1 centre point, 1 point on line
  measures "d230" diameter of A0
  measures "d231" distance from line of L2 A0.centre
extrude "Extrusion30" [suppressed]
sketch "Sketch31" plane through (-128.905, 3.175, 135.400264) normal (0, 0, -1) x (-1, 0, 0)
  line L0 (0, 0) -> (20.32, 0) projected
  line L1 (0, 0) -> (0, 20.32) projected
  line L2 (20.32, 20.32) -> (0, 20.32) projected
  line L3 (20.32, 0) -> (20.32, 20.32) projected
  circle A0 centre (6.35, 17.145) radius 1.5875
  point P0 (-128.905, -3.175)
  dimension "d234" = 3.175
  dimension "d235" = 3.175
  dimension "d236" = 6.35
  constraints: 1 centre point
  measures "d234" diameter of A0
  measures "d235" distance from line of L2 A0.centre
  measures "d236" distance from line of L1 A0.centre
extrude "Extrusion31" [suppressed]
fillet "Fillet5" [suppressed]
fillet "Fillet6" [suppressed]
sketch "Sketch32" plane through (-207.790264, 3.175, 44.45) normal (0, 1, 0) x (1, 0, 0)
  circle A0 centre (63.645264, -95.6945) radius 2.54
  circle A1 centre (128.542264, -95.6945) radius 2.54
  circle A2 centre (128.542264, -12.2555) radius 2.54
  circle A3 centre (63.645264, -12.2555) radius 2.54
  line L0 (58.565264, -107.95) -> (58.565264, 0)
  line L1 (84.727264, 12.210264) -> (102.253264, 12.210264)
  line L2 (55.390264, -3.175) -> (55.390264, -104.775)
  line L3 (55.390264, -53.975) -> (199.680527, -53.975) construction
  line L4 (207.790264, 44.45) -> (207.790264, -152.4)
  line L5 (133.005527, 33.165264) -> (183.805527, 33.165264)
  line L6 (183.805527, 33.165264) -> (183.805527, 11.575264)
  line L7 (183.805527, 11.575264) -> (133.005527, 11.575264)
  line L8 (133.005527, 11.575264) -> (133.005527, 33.165264)
  line L9 (133.005527, -119.525264) -> (183.805527, -119.525264)
  line L10 (183.805527, -119.525264) -> (183.805527, -141.115264)
  line L11 (183.805527, -141.115264) -> (133.005527, -141.115264)
  line L12 (133.005527, -141.115264) -> (133.005527, -119.525264)
  line L13 (144.892727, -46.336736) -> (144.892727, 9.670264)
  line L14 (144.892727, 9.670264) -> (185.532727, 9.670264)
  line L15 (185.532727, 9.670264) -> (185.532727, -46.336736)
  line L16 (185.532727, -46.336736) -> (144.892727, -46.336736)
  line L17 (144.892727, -117.620264) -> (144.892727, -61.613264)
  line L18 (144.892727, -61.613264) -> (185.532727, -61.613264)
  line L19 (185.532727, -61.613264) -> (185.532727, -117.620264)
  line L20 (185.532727, -117.620264) -> (144.892727, -117.620264)
  line L21 (58.565264, 0) -> (58.565264, -107.95)
  line L22 (58.565264, -107.95) -> (0, -107.95)
  line L23 (0, -107.95) -> (0, -130.193109)
  line L24 (0, -130.193109) -> (56.388618, -144.290264)
  line L25 (56.388618, -144.290264) -> (84.727264, -144.290264)
  line L26 (84.727264, -144.290264) -> (84.727264, -141.115264)
  line L27 (84.727264, -141.115264) -> (68.090264, -141.115264)
  line L28 (68.090264, -141.115264) -> (68.090264, -130.320264)
  line L29 (68.090264, -130.320264) -> (84.727264, -130.320264)
  line L30 (84.727264, -130.320264) -> (84.727264, -120.160264)
  line L31 (84.727264, -120.160264) -> (102.253264, -120.160264)
  line L32 (102.253264, -120.160264) -> (102.253264, -130.320264)
  line L33 (102.253264, -130.320264) -> (118.890264, -130.320264)
  line L34 (118.890264, -130.320264) -> (118.890264, -141.115264)
  line L35 (118.890264, -141.115264) -> (102.253264, -141.115264)
  line L36 (102.253264, -141.115264) -> (102.253264, -144.290264)
  line L37 (102.253264, -144.290264) -> (199.680527, -144.290264)
  line L38 (199.680527, -144.290264) -> (199.680527, 36.340264)
  line L39 (199.680527, 36.340264) -> (102.253264, 36.340264)
  line L40 (102.253264, 36.340264) -> (102.253264, 33.165264)
  line L41 (102.253264, 33.165264) -> (118.890264, 33.165264)
  line L42 (118.890264, 33.165264) -> (118.890264, 22.370264)
  line L43 (118.890264, 22.370264) -> (102.253264, 22.370264)
  line L44 (102.253264, 22.370264) -> (102.253264, 12.210264)
  line L45 (102.253264, 12.210264) -> (84.727264, 12.210264)
  line L46 (84.727264, 12.210264) -> (84.727264, 22.370264)
  line L47 (84.727264, 22.370264) -> (68.090264, 22.370264)
  line L48 (68.090264, 22.370264) -> (68.090264, 33.165264)
  line L49 (68.090264, 33.165264) -> (84.727264, 33.165264)
  line L50 (84.727264, 33.165264) -> (84.727264, 36.340264)
  line L51 (84.727264, 36.340264) -> (56.388618, 36.340264)
  line L52 (56.388618, 36.340264) -> (36.467264, 31.359925)
  line L53 (36.467264, 31.359925) -> (36.467264, 24.13)
  line L54 (36.467264, 24.13) -> (7.547563, 24.13)
  line L55 (7.547563, 24.13) -> (0, 22.243109)
  line L56 (0, 22.243109) -> (0, 0)
  line L57 (0, 0) -> (58.565264, 0)
  dimension "d241" = 5.08
  dimension "d242" = 83.439
  dimension "d243" = 64.897
  dimension "d244" = 5.08
  dimension "d307" = 41.7195
  constraints: 4 centre point, 3 equal radius, 2 end point, 2 horizontal alignment, 2 midpoint, 2 vertical alignment, 1 perpendicular
  measures "d241" diameter of A2
  measures "d242" distance of A0.centre A3.centre
  measures "d243" distance of A2.centre A3.centre
  measures "d244" distance from line of L0 A0.centre
  measures "d307" distance from line of L3 A3.centre
extrude "Extrusion32" add sketch "Sketch32" along normal blind 31.75 contours A0 | A1 | A2 | A3
sketch "Sketch33" plane through (0, 40.64, 196.85) normal (1, 0, 0) x (0, 0, -1)
  line L0 (91.821, -15.24) -> (105.029, -15.24)
  line L1 (105.029, -15.24) -> (105.029, -21.59)
  line L2 (105.029, -21.59) -> (91.821, -21.59)
  line L3 (91.821, -21.59) -> (91.821, -15.24)
  circle A0 centre (98.425, -10.16) radius 2.54
  line L4 (152.4, 6.985) -> (44.45, 6.985) projected
  line L5 (98.425, 6.985) -> (98.425, -40.64) construction
  line L6 (149.225, -40.64) -> (47.625, -40.64) projected
  circle A1 centre (84.455, -18.415) radius 1.905
  circle A2 centre (112.395, -18.415) radius 1.905
  line L7 (82.55, -18.415) -> (114.3, -18.415) construction
  point P0 (196.85, -40.64)
  point P1 (105.029, -18.415)
  point P2 (98.425, -18.415)
  point P3 (91.821, -18.415)
  dimension "d254" = 3.81
  dimension "d248" = 13.208
  dimension "d249" = 6.604
  dimension "d250" = 5.08
  dimension "d251" = 5.08
  dimension "d252" = 6.35
  dimension "d253" = 19.05
  dimension "d255" = 31.75
  constraints: 12 end point, 6 point on line, 5 midpoint, 2 horizontal alignment, 2 parallel, 1 centre point, 1 horizontal, 1 perpendicular, 4 other
  measures "d248" distance between parallel lines of L3 L1
  measures "d249" distance between parallel lines of L5 L3
  measures "d250" diameter of A0
  measures "d251" distance from line of L0 A0.centre
  measures "d252" distance between parallel lines of L2 L0
  measures "d253" distance between parallel lines of L6 L2
  measures "d255" distance of L7.end L7.start
extrude "Extrusion33" cut sketch "Sketch33" against normal up to surface (3.175 mm away)
sketch "Sketch34" plane through (-79.248, 34.925, 140.1445) normal (0, 1, 0) x (1, 0, 0)
  circle A0 centre (0, 83.439) radius 2.54
  circle A1 centre (0, 83.439) radius 2.54
  circle A2 centre (0, 0) radius 2.54
  circle A3 centre (-64.897, 83.439) radius 2.54
  circle A4 centre (-64.897, 0) radius 2.54
  line L0 (4.463264, 128.859764) -> (55.263264, 128.859764)
  line L1 (55.263264, 128.859764) -> (55.263264, 107.269764)
  line L2 (55.263264, 107.269764) -> (4.463264, 107.269764)
  line L3 (4.463264, 107.269764) -> (4.463264, 128.859764)
  line L4 (4.463264, -23.830764) -> (55.263264, -23.830764)
  line L5 (55.263264, -23.830764) -> (55.263264, -45.420764)
  line L6 (55.263264, -45.420764) -> (4.463264, -45.420764)
  line L7 (4.463264, -45.420764) -> (4.463264, -23.830764)
  line L8 (16.350464, 49.357764) -> (16.350464, 105.364764)
  line L9 (16.350464, 105.364764) -> (56.990464, 105.364764)
  line L10 (56.990464, 105.364764) -> (56.990464, 49.357764)
  line L11 (56.990464, 49.357764) -> (16.350464, 49.357764)
  line L12 (16.350464, -21.925764) -> (16.350464, 34.081236)
  line L13 (16.350464, 34.081236) -> (56.990464, 34.081236)
  line L14 (56.990464, 34.081236) -> (56.990464, -21.925764)
  line L15 (56.990464, -21.925764) -> (16.350464, -21.925764)
  line L16 (-69.977, 95.6945) -> (-69.977, -12.2555)
  line L17 (-69.977, -12.2555) -> (-128.542264, -12.2555)
  line L18 (-128.542264, -12.2555) -> (-128.542264, -34.498609)
  line L19 (-128.542264, -34.498609) -> (-72.153646, -48.595764)
  line L20 (-72.153646, -48.595764) -> (-43.815, -48.595764)
  line L21 (-43.815, -48.595764) -> (-43.815, -45.420764)
  line L22 (-43.815, -45.420764) -> (-60.452, -45.420764)
  line L23 (-60.452, -45.420764) -> (-60.452, -34.625764)
  line L24 (-60.452, -34.625764) -> (-43.815, -34.625764)
  line L25 (-43.815, -34.625764) -> (-43.815, -24.465764)
  line L26 (-43.815, -24.465764) -> (-26.289, -24.465764)
  line L27 (-26.289, -24.465764) -> (-26.289, -34.625764)
  line L28 (-26.289, -34.625764) -> (-9.652, -34.625764)
  line L29 (-9.652, -34.625764) -> (-9.652, -45.420764)
  line L30 (-9.652, -45.420764) -> (-26.289, -45.420764)
  line L31 (-26.289, -45.420764) -> (-26.289, -48.595764)
  line L32 (-26.289, -48.595764) -> (71.138264, -48.595764)
  line L33 (71.138264, -48.595764) -> (71.138264, 132.034764)
  line L34 (71.138264, 132.034764) -> (-26.289, 132.034764)
  line L35 (-26.289, 132.034764) -> (-26.289, 128.859764)
  line L36 (-26.289, 128.859764) -> (-9.652, 128.859764)
  line L37 (-9.652, 128.859764) -> (-9.652, 118.064764)
  line L38 (-9.652, 118.064764) -> (-26.289, 118.064764)
  line L39 (-26.289, 118.064764) -> (-26.289, 107.904764)
  line L40 (-26.289, 107.904764) -> (-43.815, 107.904764)
  line L41 (-43.815, 107.904764) -> (-43.815, 118.064764)
  line L42 (-43.815, 118.064764) -> (-60.452, 118.064764)
  line L43 (-60.452, 118.064764) -> (-60.452, 128.859764)
  line L44 (-60.452, 128.859764) -> (-43.815, 128.859764)
  line L45 (-43.815, 128.859764) -> (-43.815, 132.034764)
  line L46 (-43.815, 132.034764) -> (-72.153646, 132.034764)
  line L47 (-72.153646, 132.034764) -> (-92.075, 127.054425)
  line L48 (-92.075, 127.054425) -> (-92.075, 119.8245)
  line L49 (-92.075, 119.8245) -> (-120.994701, 119.8245)
  line L50 (-120.994701, 119.8245) -> (-128.542264, 117.937609)
  line L51 (-128.542264, 117.937609) -> (-128.542264, 95.6945)
  line L52 (-128.542264, 95.6945) -> (-69.977, 95.6945)
  circle A5 centre (0, 83.439) radius 1.5875
  circle A6 centre (0, 0) radius 1.5875
  circle A7 centre (-64.897, 0) radius 1.5875
  circle A8 centre (-64.897, 83.439) radius 1.5875
  point P0 (79.248, 140.1445)
  dimension "d261" = 3.175
  dimension "d262" = 3.175
  dimension "d263" = 3.175
  dimension "d264" = 3.175
  constraints: 4 centre point, 4 coincident
  measures "d261" diameter of A5
  measures "d262" diameter of A6
  measures "d263" diameter of A7
  measures "d264" diameter of A8
extrude "Extrusion34" cut sketch "Sketch34" against normal up to surface (31.75 mm away) contours A5 | A6 | A7 | A8
fillet "Fillet7" radius 3.175 4 edges at (-105.537, 33.02, 7.2299) (-123.063, 33.02, 7.2299) (-123.063, 33.02, 27.1597) (-105.537, 33.02, 27.1597)
fillet "Fillet8" radius 3.175 4 edges at (-105.537, 33.02, 189.6201) (-123.063, 33.02, 189.6201) (-105.537, 33.02, 169.6903) (-123.063, 33.02, 169.6903)